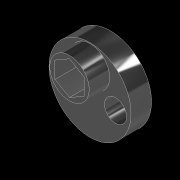
# Autodesk Inventor part: ShufflerMidCam
Saved by Autodesk Inventor 2022 (Build 260153000, 153)
## iProperties
Created: 2022-03-06
Part Number: ShufflerMidCam
Material: Custom TPU
Document SubType Name: Modeling
Designer: tandu
Density: 1.21 g/cm^3
Appearance: Smoked - Light
Author: tandu
Autodesk Inventor part; units mm, degrees
ref_plane "YZ Plane" through (0, 0, 0) normal (1, 0, 0) x (0, 1, 0)
ref_plane "XZ Plane" through (0, 0, 0) normal (0, 1, 0) x (-1, 0, 0)
ref_plane "XY Plane" through (0, 0, 0) normal (0, 0, 1) x (1, 0, 0)
sketch "Sketch1" plane through (0, 0, 0) normal (0, 0, 1) x (1, 0, 0)
  line L0 (27.0399, -21.1099) -> (29.2899, -19.8109)
  line L1 (27.0399, -23.708) -> (27.0399, -21.1099)
  line L2 (29.2899, -19.8109) -> (31.5399, -21.1099)
  line L3 (31.5399, -21.1099) -> (31.5399, -23.708)
  line L4 (29.2899, -25.007) -> (27.0399, -23.708)
  line L5 (31.5399, -23.708) -> (29.2899, -25.007)
  line L6 (31.5399, -23.708) -> (27.0399, -21.1099) construction
  line L7 (31.5399, -21.1099) -> (27.0399, -23.708) construction
  line L8 (29.2899, -25.007) -> (29.2899, -19.8109) construction
  line L9 (-2.25, 1.299) -> (0, 2.5981)
  line L10 (-2.25, -1.299) -> (-2.25, 1.299)
  line L11 (0, 2.5981) -> (2.25, 1.299)
  line L12 (2.25, 1.299) -> (2.25, -1.299)
  line L13 (0, -2.5981) -> (-2.25, -1.299)
  line L14 (2.25, -1.299) -> (0, -2.5981)
  line L15 (2.25, -1.299) -> (-2.25, 1.299) construction
  line L16 (2.25, 1.299) -> (-2.25, -1.299) construction
  line L17 (0, -2.5981) -> (0, 2.5981) construction
  line L18 (0, 0) -> (5.6649, 0) construction
  line L19 (0, 0) -> (3.9513, -3.9513) construction
  circle A0 centre (3.9513, -3.9513) radius 1.7145
  circle A1 centre (0, -3.175) radius 6.35
  line L20 (0, -3.175) -> (0, 0) construction
  line L21 (0, 0) -> (-3.9513, -3.9513) construction
  circle A2 centre (-3.9513, -3.9513) radius 1.7145
  circle A3 centre (0, 0) radius 3.048
  point P0 (29.2899, -22.4089)
  dimension "d2" = 60
  dimension "d3" = 4.5
  dimension "d4" = 60
  dimension "d5" = 4.5
  dimension "d7" = 45
  dimension "d8" = 5.588
  dimension "d9" = 3.429
  dimension "d10" = 12.7
  dimension "d11" = 3.175
  dimension "d12" = 45
  dimension "d18" = 6.096
  constraints: 44 end point, 11 equal length, 5 vertical, 4 centre point, 4 coincident, 4 horizontal alignment, 4 parallel, 2 midpoint, 2 vertical alignment, 1 equal radius, 1 horizontal
  measures "d2" angle of L3 L2
  measures "d3" distance between parallel lines of L1 L3
  measures "d4" angle of L12 L11
  measures "d5" distance between parallel lines of L10 L12
  measures "d7" angle of L18 L19
  measures "d8" distance of L18.start L19.end
  measures "d9" diameter of A0
  measures "d10" diameter of A1
  measures "d11" distance of L20.start L18.start
  measures "d12" angle of L17 L21
  measures "d18" diameter of A3
extrude "Base" add sketch "Sketch1" along normal blind 3.175 contours A1 | A2 | A3
extrude "Extrusion3" add sketch "Sketch1" along normal blind 3.175 from surface at 3.175 contours A3
equation "\"d7\" = NubAngle"
equation "\"d10\" = CamSize"
equation "\"d11\" = Offset"
equation "\"d12\" = NubAngle"
equation "\"NubAngle\" = 45deg"
equation "\"CamSize\" = 12.7"
equation "\"Offset\" = 3.175"
body "Solid1"
